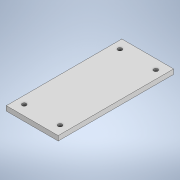
# Autodesk Inventor part: plate4atrduino
Saved by Autodesk Inventor 2022 (Build 260153000, 153)
## iProperties
Created: 2021-09-28
Part Number: plate4atrduino
Material: Generic
Document SubType Name: Modeling
Designer: royja
Density: 1 g/cm^3
Appearance: Default
Author: royja
Autodesk Inventor part; units mm, degrees
ref_plane "YZ Plane" through (0, 0, 0) normal (1, 0, 0) x (0, 1, 0)
ref_plane "XZ Plane" through (0, 0, 0) normal (0, 1, 0) x (-1, 0, 0)
ref_plane "XY Plane" through (0, 0, 0) normal (0, 0, 1) x (1, 0, 0)
sketch "Sketch1" plane through (0, 0, 0) normal (0, 1, 0) x (-1, 0, 0)
  line L0 (0, 0) -> (22, 0)
  line L1 (22, 0) -> (22, -49)
  line L2 (22, -49) -> (0, -49)
  line L3 (0, -49) -> (0, 0)
  dimension "d0" = 22
  dimension "d1" = 49
  constraints: 8 end point, 2 parallel, 1 horizontal, 1 perpendicular
  measures "d0" distance of L1.end L2.end
  measures "d1" distance of L0.end L1.end
extrude "Extrusion1" add sketch "Sketch1" along normal blind 2
sketch "Sketch2" plane through (0, 2, 0) normal (0, 1, 0) x (1, 0, 0)
  line L0 (-22, 0) -> (0, 0) projected
  line L1 (0, 0) -> (0, 49) projected
  line L2 (-18.62, 44.82) -> (-3.38, 44.82) construction
  line L3 (-3.38, 44.82) -> (-3.38, 4.18) construction
  line L4 (-3.38, 4.18) -> (-18.62, 4.18) construction
  line L5 (-18.62, 4.18) -> (-18.62, 44.82) construction
  line L6 (-18.62, 44.82) -> (-3.38, 4.18) construction
  line L7 (-3.38, 44.82) -> (-18.62, 4.18) construction
  circle A0 centre (-18.62, 4.18) radius 0.885
  circle A1 centre (-18.62, 44.82) radius 0.885
  circle A2 centre (-3.38, 44.82) radius 0.885
  circle A3 centre (-3.38, 4.18) radius 0.885
  point P0 (0, 24.5)
  point P1 (-11, 0)
  point P2 (-3.38, 0)
  point P3 (0, 4.18)
  point P4 (-11, 24.5)
  dimension "d4" = 11
  dimension "d5" = 7.62
  dimension "d6" = 20.32
  dimension "d8" = 1.77
  dimension "d9" = 1.77
  dimension "d10" = 1.77
  dimension "d11" = 1.77
  constraints: 12 end point, 5 coincident, 4 centre point, 3 midpoint, 2 parallel, 2 point on line, 1 horizontal, 1 perpendicular
  measures "d4" distance of L0.end point (-11, 0)
  measures "d5" distance of point (-11, 0) point (-3.38, 0)
  measures "d6" distance of point (0, 24.5) point (0, 4.18)
  measures "d8" diameter of A0
  measures "d9" diameter of A1
  measures "d10" diameter of A2
  measures "d11" diameter of A3
extrude "Extrusion2" cut sketch "Sketch2" against normal up to next
body "Solid1"
